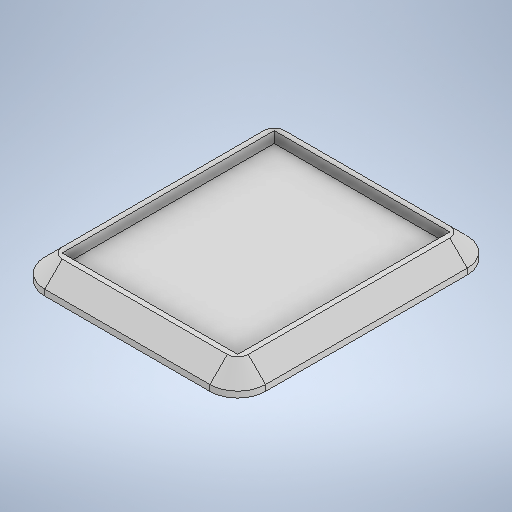
# Autodesk Inventor part: IMU_Base_T-Shirt
Saved by Autodesk Inventor 2025.2 (Build 292293000, 293)
## iProperties
Created: 2024-11-14
Part Number: IMU_Base_T-Shirt
Material: Generic
Document SubType Name: Modeling
Designer: matss
Density: 1 g/cm^3
Appearance: Default
Author: matss
Autodesk Inventor part; units mm, degrees
ref_plane "YZ Plane" through (0, 0, 0) normal (1, 0, 0) x (0, 1, 0)
ref_plane "XZ Plane" through (0, 0, 0) normal (0, 1, 0) x (-1, 0, 0)
ref_plane "XY Plane" through (0, 0, 0) normal (0, 0, 1) x (1, 0, 0)
sketch "Sketch1" plane through (0, 0, 0) normal (0, 1, 0) x (-1, 0, 0)
  line L0 (31.75, 37) -> (-31.75, 37)
  line L1 (-31.75, 37) -> (-31.75, -37)
  line L2 (-31.75, -37) -> (31.75, -37)
  line L3 (31.75, -37) -> (31.75, 37)
  point P0 (0, 0)
  point P1 (31.75, 0)
  point P2 (0, 37)
  dimension "d0" = 74
  dimension "d1" = 63.5
  constraints: 8 end point, 2 midpoint, 2 parallel, 1 horizontal, 1 horizontal alignment, 1 perpendicular, 1 vertical alignment
  measures "d0" distance of L2.end L0.start
  measures "d1" distance of L0.start L0.end
extrude "Extrusion1" add sketch "Sketch1" along normal blind 0.96
sketch "Sketch2" plane through (0, 0.96, 0) normal (0, 1, 0) x (1, 0, 0)
  line L0 (31.75, -37) -> (31.75, 37) projected
  line L1 (31.75, 37) -> (-31.75, 37) projected
  line L2 (-31.75, 37) -> (-31.75, -37) projected
  line L3 (-31.75, -37) -> (31.75, -37) projected
  line L4 (-31.75, 0) -> (31.75, 0)
  line L5 (0, -37) -> (0, 37)
  circle A0 centre (-16, -16) radius 4.25
  circle A1 centre (-16, 16) radius 4.25
  circle A2 centre (16, 16) radius 4.25
  circle A3 centre (16, -16) radius 4.25
  point P0 (0, 0)
  dimension "d13" = 8.5
  dimension "d14" = 32
  dimension "d15" = 32
  constraints: 4 centre point, 4 end point, 4 midpoint, 3 equal radius, 3 other
  measures "d13" diameter of A0
  measures "d14" distance of A3.centre A0.centre
  measures "d15" distance of A1.centre A0.centre
extrude "Extrusion2" add sketch "Sketch2" along normal blind 1.92
sketch "Sketch3" plane through (0, 2.88, 0) normal (0, 1, 0) x (1, 0, 0)
  line L0 (-31.75, 37) -> (-31.75, -37) projected
  line L1 (-31.75, -37) -> (31.75, -37) projected
  line L2 (31.75, -37) -> (31.75, 37) projected
  line L3 (31.75, 37) -> (-31.75, 37) projected
  point P0 (0, 0)
extrude "Extrusion3" add sketch "Sketch3" along normal blind 0.64
fillet "Fillet1" radius 8 4 edges at (31.75, 1.76, 37) (-31.75, 1.76, 37) (-31.75, 1.76, -37) (31.75, 1.76, -37)
ref_plane "Arbeitsebene2" through (29.4069, 3.52, -34.6569) normal (-0.7625, 0, -0.647) x (0, -1, 0)
sketch "Skizze7" plane through (0, 3.52, 0) normal (0, 1, 0) x (1, 0, 0)
  line L0 (-23.75, -37) -> (23.75, -37) projected
  arc A0 (23.75, -37) -> (31.75, -29) centre (23.75, -29) ccw projected
  line L1 (31.75, -29) -> (31.75, 29) projected
  arc A1 (31.75, 29) -> (23.75, 37) centre (23.75, 29) ccw projected
  line L2 (23.75, 37) -> (-23.75, 37) projected
  arc A2 (-23.75, 37) -> (-31.75, 29) centre (-23.75, 29) ccw projected
  line L3 (-31.75, 29) -> (-31.75, -29) projected
  arc A3 (-31.75, -29) -> (-23.75, -37) centre (-23.75, -29) ccw projected
  line L4 (23.75, -37) -> (-27, -37)
  line L5 (-31.75, -29) -> (-31.75, 29)
  line L6 (-23.75, 37) -> (23.75, 37)
  line L7 (31.75, 29) -> (31.75, -29)
  arc A4 (23.75, -37) -> (31.75, -29) centre (23.75, -29) ccw
  arc A5 (-32.385, -29) -> (-27, -37) centre (-23.75, -29) ccw
  arc A6 (-23.75, 37) -> (-31.75, 29) centre (-23.75, 29) ccw
  arc A7 (31.75, 29) -> (23.75, 37) centre (23.75, 29) ccw
  point P0 (0, 0)
  constraints: 12 point on circle, 8 end point, 4 centre point, 4 coincident, 3 perpendicular, 1 point on line
extrude "Extrusion4" add sketch "Skizze7" along normal blind 3.2
sketch "Skizze8" plane through (0, 6.72, 0) normal (0, 1, 0) x (1, 0, 0)
  line L0 (25.25, 30.5) -> (-25.25, 30.5)
  line L1 (-25.25, 30.5) -> (-25.25, -30.5)
  line L2 (-25.25, -30.5) -> (25.25, -30.5)
  line L3 (25.25, -30.5) -> (25.25, 30.5)
  line L4 (25.25, 30.5) -> (-25.25, -30.5) construction
  line L5 (-25.25, 30.5) -> (25.25, -30.5) construction
  point P0 (0, 0)
  dimension "d25" = 61
  dimension "d26" = 50.5
  constraints: 12 end point, 2 midpoint, 2 parallel, 1 horizontal, 1 perpendicular
  measures "d25" distance of L0.end L1.end
  measures "d26" distance of L1.end L2.end
extrude "Extrusion5" cut sketch "Skizze8" against normal blind 3.2
chamfer "Fasen3" distance 5 angle 45 8 edges at (31.75, 6.72, 0) (29.4069, 6.72, -34.6569) (0, 6.72, -37) (-29.4069, 6.72, -34.6569) (-31.75, 6.72, 0) (-29.4069, 6.72, 34.6569) (0, 6.72, 37) (29.4069, 6.72, 34.6569)
body "Solid1"
